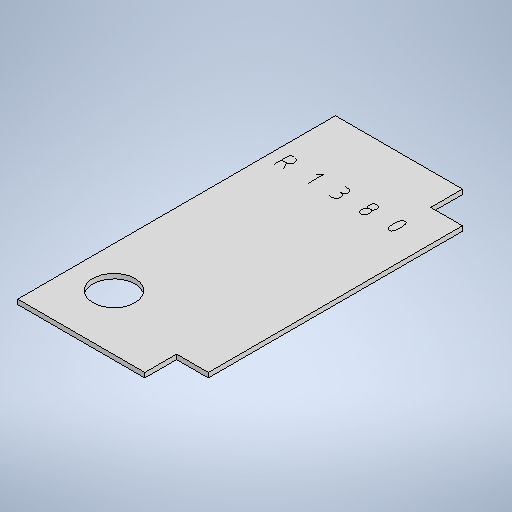
# Autodesk Inventor part: Part14
Saved by Autodesk Inventor 2025.3 (Build 293356030, 356C)
## iProperties
Created: 2026-01-14
Part Number: Part14
Material: Stainless Steel
Document SubType Name: Sheet Metal
Designer: admin
Mass: 447.548 g
Surface Area: 393.455 cm^2
Volume: 55.9434 cm^3
Density: 8 g/cm^3
Flat Pattern Width: 10 cm
Flat Pattern Length: 20 cm
Flat Pattern Area: 200 cm^2
Sheet Metal Rule: AISI304 3mm Die 32
Sheet Metal Width: 100,000 mm
Sheet Metal Length: 200,000 mm
Sheet Metal Area: 20000,000 mm^2
Appearance: Default
Author: admin
Autodesk Inventor part; units mm, degrees
ref_plane "YZ Plane" through (0, 0, 0) normal (1, 0, 0) x (0, 1, 0)
ref_plane "XZ Plane" through (0, 0, 0) normal (0, 1, 0) x (-1, 0, 0)
ref_plane "XY Plane" through (0, 0, 0) normal (0, 0, 1) x (1, 0, 0)
sketch "Sketch7" plane through (0, 0, 0) normal (0, 0, 1) x (1, 0, 0)
  line L0 (0, 0) -> (100, 0)
  line L1 (100, 0) -> (100, -200)
  line L2 (100, -200) -> (0, -200)
  line L3 (0, -200) -> (0, 0)
  line L4 (100, 0) -> (80, 0)
  line L5 (80, 0) -> (80, -20)
  line L6 (80, -20) -> (100, -20)
  line L7 (100, -20) -> (100, 0)
  line L8 (100, -200) -> (80, -200)
  line L9 (80, -200) -> (80, -180)
  line L10 (80, -180) -> (100, -180)
  line L11 (100, -180) -> (100, -200)
  dimension "d23" = 100
  dimension "d24" = 200
  dimension "d25" = 20
  dimension "d26" = 20
  measures "d23" distance of L1.end L2.end
  measures "d24" distance of L0.end L1.end
  measures "d25" distance of L6.end L5.end
  measures "d26" distance of L5.end L4.end
extrude "Plate3" add sketch "Sketch7" along normal blind 3 contours L0 L5 L6 L1 L10 L9 L2 L3
sketch "Sketch8" plane through (0, 0, 3) normal (0, 0, 1) x (1, 0, 0)
  line L0 (6.2166, -35.2952) -> (70.6562, -35.2952) construction
  line L1 (70.6562, -35.2952) -> (70.6562, -48.8117) construction
  line L2 (70.6562, -48.8117) -> (6.2166, -48.8117) construction
  line L3 (6.2166, -48.8117) -> (6.2166, -35.2952) construction
  point P0 (0, 0)
  constraints: 2 other
mark "Mark2"
sketch "Sketch9" plane through (0, -200, 3) normal (0, 0, 1) x (1, 0, 0)
  circle A0 centre (25.6213, 34.9394) radius 13.2577
  point P0 (0, 200)
  constraints: 1 centre point
extrude "Cut1" cut sketch "Sketch9" against normal blind 3
equation "\"d28\" = Thickness"
equation "\"d27\" = Thickness"
equation "\"BendReliefWidth\" = Thickness"
equation "\"BendReliefDepth\" = 0.5 * Thickness"
equation "\"CornerReliefSize\" = 4 * Thickness"
equation "\"MinimumRemnant\" = 2 * Thickness"
equation "\"TransitionRadius\" = BendRadius"
equation "\"JacobiRadiusSize\" = BendRadius"
equation "\"GapSize\" = Thickness"
equation "\"Thickness\" = 3"
equation "\"BendRadius\" = 5"
body "Solid2"
